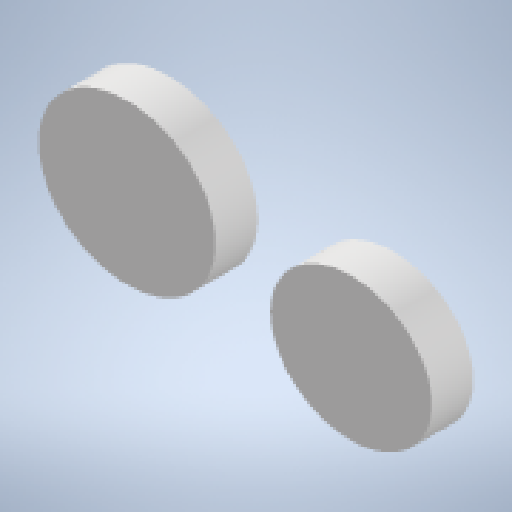
# Autodesk Inventor part: HandsPeach
Saved by Autodesk Inventor 2023 (Build 270158000, 158)
## iProperties
Created: 2022-11-09
Part Number: HandsPeach
Material: Generic
Document SubType Name: Modeling
Designer: reide
Density: 1 g/cm^3
Appearance: Default
Author: reide
Autodesk Inventor part; units mm, degrees
ref_plane "YZ Plane" through (0, 0, 0) normal (1, 0, 0) x (0, 1, 0)
ref_plane "XZ Plane" through (0, 0, 0) normal (0, 1, 0) x (-1, 0, 0)
ref_plane "XY Plane" through (0, 0, 0) normal (0, 0, 1) x (1, 0, 0)
sketch "Sketch1" plane through (0, 0, 0) normal (0, 0, 1) x (1, 0, 0)
  arc A0 (-0.9046, 4.9369) -> (-5.1014, 1.0558) centre (0, -0.2509) ccw projected
  ellipse E0 centre (-9.8648, 1.4867) end of major axis (-14.6282, 1.9177) minor radius 4.1297 (-5.2276, 0.3848) -> (-5.1014, 1.0558) ccw projected
  arc A1 (-5.1014, 1.0558) -> (-5.2276, 0.3848) centre (0, -0.2509) ccw projected
  ellipse E1 centre (-9.8648, 1.4867) end of major axis (-5.1014, 1.0558) minor radius 4.1297 (-5.1014, 1.0558) -> (-7.337, 4.9369) ccw projected
  line L0 (-0.9046, 4.9369) -> (-7.337, 4.9369) projected
  arc A2 (-59.5755, 4.9369) -> (-60.9121, 2.898) centre (-42.2911, -7.8518) ccw projected
  spline S0 degree 3 poles (-56.8976, 1.1787) (-56.9052, 1.1498) (-56.9132, 1.121) (-57.0437, 0.6744) (-57.2476, 0.2806) (-57.7298, -0.3295) (-57.9833, -0.5662) (-58.5274, -0.9213) (-58.8121, -1.0494) (-59.3678, -1.1788) (-59.635, -1.195) (-60.058, -1.1328) (-60.2177, -1.0876) (-60.3681, -1.0211) (-60.6523, -0.8955) (-60.9006, -0.6925) (-61.1923, -0.3032) (-61.2786, -0.1486) (-61.5034, 0.3943) (-61.5565, 0.8142) (-61.4866, 1.7511) (-61.3117, 2.265) (-60.9956, 2.7766) (-60.9549, 2.838) (-60.9121, 2.898) knots -2.04297 -2.04297 -2.04297 -2.04297 -2.033998 -2.033998 -1.903383 -1.903383 -1.8007 -1.8007 -1.70847 -1.70847 -1.629539 -1.629539 -1.580207 -1.580207 -1.580207 -1.486994 -1.486994 -1.434286 -1.434286 -1.31073 -1.31073 -1.152429 -1.152429 -1.130329 -1.130329 -1.130329 -1.130329 projected
  arc A3 (-54.0351, 4.9369) -> (-56.8976, 1.1787) centre (-49.1589, -1.7464) ccw projected
  line L1 (-48.7905, 4.9369) -> (-54.0351, 4.9369) projected
  arc A4 (-48.7905, 4.9369) -> (-44.3601, 1.1398) centre (-35.3577, 16.1268) ccw projected
  arc A5 (-44.3601, 1.1398) -> (-53.317, -6.887) centre (-40.9405, -11.6869) ccw projected
  arc A6 (-53.317, -6.887) -> (-55.157, -23.9352) centre (-25.4946, -18.5133) ccw projected
  arc A7 (-55.157, -23.9352) -> (-62.1701, -35.1777) centre (-44.1446, -38.6133) ccw projected
  arc A8 (-62.1701, -35.1777) -> (-48.8402, -39.4479) centre (-51.2446, -24.0133) ccw projected
  arc A9 (-48.8402, -39.4479) -> (-3.2686, -48.1109) centre (-20.7238, -15.7377) ccw projected
  arc A10 (-3.2686, -48.1109) -> (9.8317, -48.8006) centre (4.081, -33.2699) ccw projected
  arc A11 (9.8317, -48.8006) -> (7.0355, -38.6809) centre (-4.7854, -47.3934) ccw projected
  arc A12 (7.0355, -38.6809) -> (9.7106, -25.1352) centre (-12.1725, -27.8505) ccw projected
  arc A13 (9.7106, -25.1352) -> (3.1866, -3.0874) centre (0, -16.0194) ccw projected
  arc A14 (3.1866, -3.0874) -> (0.8135, 3.9369) centre (0, -0.2509) ccw projected
  line L2 (0.8135, 3.9369) -> (2.1928, 3.9369) projected
  arc A15 (3.1928, 4.9369) -> (2.1928, 3.9369) centre (3.1928, 3.9369) ccw projected
  line L3 (70.356, 4.9369) -> (3.1928, 4.9369) projected
  line L4 (70.356, 12.9385) -> (70.356, 4.9369) projected
  line L5 (-61.4202, 12.9385) -> (70.356, 12.9385) projected
  arc A16 (-63.4202, 14.9385) -> (-61.4202, 12.9385) centre (-61.4202, 14.9385) ccw projected
  line L6 (-63.4202, 107.9369) -> (-63.4202, 14.9385) projected
  arc A17 (-61.4202, 109.9369) -> (-63.4202, 107.9369) centre (-61.4202, 107.9369) ccw projected
  line L7 (70.356, 109.9369) -> (-61.4202, 109.9369) projected
  line L8 (70.356, 117.9369) -> (70.356, 109.9369) projected
  line L9 (-66.8452, 117.9369) -> (70.356, 117.9369) projected
  arc A18 (-66.8452, 117.9369) -> (-70.8452, 113.9369) centre (-66.8452, 113.9369) ccw projected
  line L10 (-70.8452, 8.9369) -> (-70.8452, 113.9369) projected
  arc A19 (-70.8452, 8.9369) -> (-66.8452, 4.9369) centre (-66.8452, 8.9369) ccw projected
  line L11 (-59.5755, 4.9369) -> (-66.8452, 4.9369) projected
  ellipse E2 centre (-10.6588, 1.4867) end of major axis (-15.0966, 1.4867) minor radius 3.9921 projected
  ellipse E3 centre (-27.2446, -17.5631) end of major axis (-30.2446, -17.5631) minor radius 2.4928 projected
  arc A20 (-54.4264, -25.7115) -> (-49.8152, -37.5715) centre (85.6711, 21.9314) ccw projected
  arc A21 (-59.946, -34.3231) -> (-49.8152, -37.5715) centre (-49.2751, -18.4657) ccw projected
  arc A22 (-54.4264, -25.7115) -> (-59.946, -34.3231) centre (-41.409, -40.1296) ccw projected
  arc A23 (-5.6405, -20.531) -> (-7.2446, -21.5631) centre (-5.8688, -21.9389) ccw projected
  arc A24 (-7.2446, -21.5631) -> (-9.1707, -19.5887) centre (-10.2446, -22.5631) ccw projected
  ellipse E4 centre (-7.4005, -19.5631) end of major axis (-7.4005, -10.5631) minor radius 1.7702 (-5.6405, -20.531) -> (-9.1707, -19.5887) ccw projected
  circle A25 centre (1.7554, -24.0133) radius 2.7388 projected
  circle A26 centre (-20.2446, -22.5631) radius 2.8284 projected
  arc A27 (0.9328, -47.5617) -> (7.225, -41.7583) centre (-13.3979, -25.7115) ccw projected
  arc A28 (7.6831, -47.4803) -> (7.225, -41.7583) centre (-10.5104, -46.0577) ccw projected
  arc A29 (0.9328, -47.5617) -> (7.6831, -47.4803) centre (4.1217, -32.0801) ccw projected
  ellipse E5 centre (0, 0) end of major axis (4.0186, -0.2759) minor radius 3.5714 projected
  ellipse E6 centre (8.2115, -20.8216) end of major axis (5.68, -20.8216) minor radius 2.1289 projected
  ellipse E7 centre (-10.6588, 1.4867) end of major axis (-6.4428, 1.4867) minor radius 3.7925
  ellipse E8 centre (0, 0) end of major axis (0, 3.3946) minor radius 3.8291
  constraints: 2 coincident, 1 centre point, 10 other
extrude "Extrusion1" add sketch "Sketch1" along normal blind 2 contours E7 | E8
body "Solid1"
